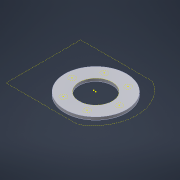
# Autodesk Inventor part: P025-Joint_carter_arbre
Saved by Autodesk Inventor 2021.3 (Build 253353000, 353)
## iProperties
Created: 2022-06-11
Part Number: P025-Joint_carter_arbre
Material: Polytetrafluoroethylene
Document SubType Name: Modeling
Designer: Rémi Heredero
Density: 2.02 g/cm^3
Appearance: PTFE
Author: Rémi Heredero
Autodesk Inventor part; units mm, degrees
ref_plane "YZ Plane" through (0, 0, 0) normal (1, 0, 0) x (0, 1, 0)
ref_plane "XZ Plane" through (0, 0, 0) normal (0, 1, 0) x (-1, 0, 0)
ref_plane "XY Plane" through (0, 0, 0) normal (0, 0, 1) x (1, 0, 0)
sketch "Sketch2" plane through (0, 0, 0) normal (0, 0, 1) x (1, 0, 0)
  circle A0 centre (0, 0) radius 11.5
  circle A1 centre (0, 0) radius 21.5
  dimension "d0" = 23
  dimension "d1" = 10
  constraints: 2 centre point, 2 coincident
  measures "d0" diameter of A0
  measures "d1" radial gap between concentric circles of A1 A0
extrude "Extrusion1" add sketch "Sketch2" along normal blind 2
sketch "Sketch3" plane through (0, 0, 2) normal (0, 0, 1) x (1, 0, 0)
  circle A0 centre (8.25, -14.2894) radius 2.25 construction
  circle A1 centre (8.25, 14.2894) radius 2.25 construction
  circle A2 centre (-16.5, 0) radius 2.25 construction
  circle A3 centre (-8.25, 14.2894) radius 2.25 construction
  circle A4 centre (16.5, 0) radius 2.25 construction
  circle A5 centre (-8.25, -14.2894) radius 2.25 construction
  circle A6 centre (0, 0) radius 11.5 construction
  arc A7 (13.4666, -26) -> (13.4666, 26) centre (-1.5, 0) ccw construction
  line L0 (-36.5, 26) -> (13.4666, 26) construction
  line L1 (-36.5, -26) -> (-36.5, 26) construction
  line L2 (13.4666, -26) -> (-36.5, -26) construction
  point P0 (0, 0)
body "Solid1"
